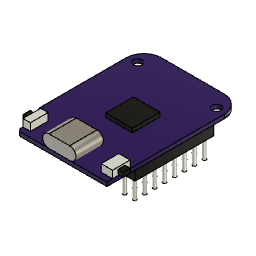
MLH1 v1.0 (Autodesk Fusion 360 archive; units mm, degrees)
design "ESP32-S2-mini"
Autodesk Fusion 360 part; units mm, degrees
sketch "Esquisse1" plane through (0, 0, 0) normal (0, 0, 1) x (1, 0, 0) in component "ESP32 S2-mini"
  line L0 (13.4, -16.1) -> (-11.6, -16.1)
  line L1 (-11.6, -16.1) -> (-11.6, 18.3)
  line L2 (-11.6, 18.3) -> (13.4, 18.3)
  line L3 (13.4, 18.3) -> (13.4, -16.1)
  line L4 (-11.6, -8.4281) -> (-9.4567, -9.7933)
  line L5 (-9.4567, -9.7933) -> (-9.4567, -15.5)
  line L6 (-9.4567, -15.5) -> (-8.8896, -16.1)
  circle A0 centre (-7.1, 13.8) radius 4.5
  circle A1 centre (8.9, 13.8) radius 4.5
  circle A2 centre (-9.1309, 14.2904) radius 1.122
  circle A3 centre (11.0247, 14.2904) radius 1.1083
  line L7 (-11.6, 11.162) -> (-6.6, 11.162)
  line L8 (-6.6, 11.162) -> (-6.6, -8.938)
  line L9 (-6.6, -8.938) -> (-11.6, -8.938)
  line L10 (-11.6, -8.938) -> (-11.6, 11.162)
  line L11 (13.4, 11.162) -> (8.4, 11.162)
  line L12 (8.4, 11.162) -> (8.4, -8.938)
  line L13 (8.4, -8.938) -> (13.4, -8.938)
  line L14 (13.4, -8.938) -> (13.4, 11.162)
  circle A4 centre (-10.5, 9.8) radius 0.4445
  circle A5 centre (-7.96, 9.8) radius 0.4445
  circle A6 centre (-10.5, 7.26) radius 0.4445
  circle A7 centre (-7.96, 7.26) radius 0.4445
  circle A8 centre (-10.5, 4.72) radius 0.4445
  circle A9 centre (-7.96, 4.72) radius 0.4445
  circle A10 centre (-10.5, 2.18) radius 0.4445
  circle A11 centre (-7.96, 2.18) radius 0.4445
  circle A12 centre (-10.5, -0.36) radius 0.4445
  circle A13 centre (-7.96, -0.36) radius 0.4445
  circle A14 centre (-10.5, -2.9) radius 0.4445
  circle A15 centre (-7.96, -2.9) radius 0.4445
  circle A16 centre (-10.5, -5.44) radius 0.4445
  circle A17 centre (-7.96, -5.44) radius 0.4445
  circle A18 centre (-10.5, -7.98) radius 0.4445
  circle A19 centre (-7.96, -7.98) radius 0.4445
  circle A20 centre (9.82, 9.8) radius 0.4445
  circle A21 centre (12.36, 9.8) radius 0.4445
  circle A22 centre (9.82, 7.26) radius 0.4445
  circle A23 centre (12.36, 7.26) radius 0.4445
  circle A24 centre (9.82, 4.72) radius 0.4445
  circle A25 centre (12.36, 4.72) radius 0.4445
  circle A26 centre (9.82, 2.18) radius 0.4445
  circle A27 centre (12.36, 2.18) radius 0.4445
  circle A28 centre (9.82, -0.36) radius 0.4445
  circle A29 centre (12.36, -0.36) radius 0.4445
  circle A30 centre (9.82, -2.9) radius 0.4445
  circle A31 centre (12.36, -2.9) radius 0.4445
  circle A32 centre (9.82, -5.44) radius 0.4445
  circle A33 centre (12.36, -5.44) radius 0.4445
  circle A34 centre (9.82, -7.98) radius 0.4445
  circle A35 centre (12.36, -7.98) radius 0.4445
  dimension "d1" = 25
  dimension "d2" = 34.4
  dimension "d3" = 4.5
  dimension "d4" = 4.5
  dimension "d7" = 5
  dimension "d8" = 20.1
  dimension "d9" = 5
  dimension "d10" = 20.1
  dimension "d36" = 0.889
  dimension "d39" = 2.54
  dimension "d40" = -17.78
  dimension "d41" = 8.5
  dimension "d42" = 1.1
  dimension "d43" = 0.889
  dimension "d44" = 8.5
  dimension "d45" = 20.32
  dimension "d48" = 2.54
  dimension "d49" = -17.78
  constraint horizontal L0
  constraint vertical L1
  constraint horizontal L2
  constraint vertical L3
  constraint coincident L1 L4.start
  constraint parallel L1 L5
  constraint coincident L0 L6.end
  constraint tangent L1 A0
  constraint tangent L2 A0
  constraint tangent L2 A1
  constraint tangent L3 A1
  constraint horizontal L7
  constraint vertical L8
  constraint horizontal L9
  constraint vertical L10
  constraint coincident L1 L7.start
  constraint horizontal L11
  constraint vertical L12
  constraint horizontal L13
  constraint vertical L14
  constraint coincident L3 L11.start
  measures "d1" distance of L0.start L0.end
  measures "d2" distance of L0.start L2.end
  measures "d3" radius of A0
  measures "d4" radius of A1
  measures "d7" distance of L7.start L7.end
  measures "d8" distance of L7.start L9.end
  measures "d9" distance of L11.start L11.end
  measures "d10" distance of L11.start L13.end
  measures "d36" diameter of A4
  measures "d41" distance of L2 A4.centre
  measures "d42" distance of L1 A4.centre
  measures "d43" diameter of A20
  measures "d44" distance of L2 A20.centre
  measures "d45" distance of A4.centre A20.centre
extrude "Extrusion1" add sketch "Esquisse1" along normal blind 1 contours L0 L2 L3 L4 L5 L6 A0 A1 L8 L9 L12 L13 | L3 A1 L11 L12 L13 L14 A20 | L3 A1 L11 | A1 L11 L12 | A1 L11 L12 A20 | L1 L4 A0 L7 L8 L9 L10 A5 | A1 A20 | A1 A20 | L1 A0 L7 | A0 L7 L8 | A0 L7 L8 A5 | A0 A5 | A0 A5 | A4 | A6 | A7 | A8 | A9 | A10 | A11 | A12 | A13 | A14 | A15 | A16 | A17 | A18 | A19 | A21 | A22 | A23 | A24 | A25 | A26 | A27 | A28 | A29 | A30 | A31 | A32 | A33 | A34 | A35 makes body 1 in component "ESP32 S2-mini"
extrude "Extrusion2" add sketch "Esquisse1" against normal blind 2.4 separate body contours L3 A1 L11 L12 L13 L14 A20 | A1 L11 L12 A20 | L1 L4 A0 L7 L8 L9 L10 A5 | A1 A20 | A1 A20 | A0 L7 L8 A5 | A0 A5 | A0 A5 | A4 | A6 | A7 | A8 | A9 | A10 | A11 | A12 | A13 | A14 | A15 | A16 | A17 | A18 | A19 | A21 | A22 | A23 | A24 | A25 | A26 | A27 | A28 | A29 | A30 | A31 | A32 | A33 | A34 | A35 makes body 2 at (-8.2667, -2.068, 0) makes body 3 at (10.0667, -2.238, 0) in component "ESP32 S2-mini"
sketch "Esquisse2" plane through (0, 0, 1) normal (0, 0, 1) x (-1, 0, 0) in component "ESP32 S2-mini"
  circle A0 centre (-11.0247, -14.2904) radius 1.1083
  circle A1 centre (9.1309, -14.2904) radius 1.122
  line L0 (-13.4, 16.1) -> (-13.4, -13.8)
  arc A2 (-13.4, -13.8) -> (-8.9, -18.3) centre (-8.9, -13.8) ccw
  line L1 (-8.9, -18.3) -> (7.1, -18.3)
  arc A3 (7.1, -18.3) -> (11.6, -13.8) centre (7.1, -13.8) ccw
  line L2 (11.6, -13.8) -> (11.6, 8.4281)
  line L3 (11.6, 8.4281) -> (9.4567, 9.7933)
  line L4 (9.4567, 9.7933) -> (9.4567, 15.5)
  line L5 (9.4567, 15.5) -> (8.8896, 16.1)
  line L6 (8.8896, 16.1) -> (-13.4, 16.1)
  line L7 (3.0077, 16.1) -> (-5.4923, 16.1)
  line L8 (-5.4923, 16.1) -> (-5.4923, 9.1)
  line L9 (-5.4923, 9.1) -> (3.0077, 9.1)
  line L10 (3.0077, 9.1) -> (3.0077, 16.1)
  line L11 (9.4567, 10.1759) -> (7.5567, 10.1759)
  line L12 (7.5567, 10.1759) -> (7.5567, 14.6759)
  line L13 (7.5567, 14.6759) -> (9.4567, 14.6759)
  line L14 (9.4567, 14.6759) -> (9.4567, 10.1759)
  line L15 (-13.4, 10.1759) -> (-10.5, 10.1759)
  line L16 (-10.5, 10.1759) -> (-10.5, 14.6759)
  line L17 (-10.5, 14.6759) -> (-13.4, 14.6759)
  line L18 (-13.4, 14.6759) -> (-13.4, 10.1759)
  line L19 (9.4567, 11.497) -> (10.8067, 11.497)
  line L20 (10.8067, 11.497) -> (10.8067, 13.297)
  line L21 (10.8067, 13.297) -> (9.4567, 13.297)
  line L22 (9.4567, 13.297) -> (9.4567, 11.497)
  line L23 (-13.4, 11.5) -> (-14.75, 11.5)
  line L24 (-14.75, 11.5) -> (-14.75, 13.3)
  line L25 (-14.75, 13.3) -> (-13.4, 13.3)
  line L26 (-13.4, 13.3) -> (-13.4, 11.5)
  line L27 (-5.7592, -5.0845) -> (1, -5.0845)
  line L28 (1, -5.0845) -> (1, 2)
  line L29 (1, 2) -> (-5.7592, 2)
  line L30 (-5.7592, 2) -> (-5.7592, -5.0845)
  dimension "d13" = 8.5
  dimension "d14" = 7
  dimension "d15" = 1.9
  dimension "d16" = 4.5
  dimension "d17" = 2.9
  dimension "d18" = 4.5
  dimension "d19" = 1.35
  dimension "d20" = 1.8
  dimension "d21" = 1.35
  dimension "d22" = 1.8
  constraint horizontal L7
  constraint vertical L8
  constraint horizontal L9
  constraint vertical L10
  constraint coincident L6 L7.start
  constraint horizontal L11
  constraint vertical L12
  constraint horizontal L13
  constraint vertical L14
  constraint coincident L4 L11.start
  constraint horizontal L15
  constraint vertical L16
  constraint horizontal L17
  constraint vertical L18
  constraint coincident L0 L15.start
  constraint horizontal L19
  constraint vertical L20
  constraint horizontal L21
  constraint vertical L22
  constraint coincident L14 L19.start
  constraint horizontal L23
  constraint vertical L24
  constraint horizontal L25
  constraint vertical L26
  constraint coincident L18 L23.start
  constraint horizontal L27
  constraint vertical L28
  constraint horizontal L29
  constraint vertical L30
  measures "d13" distance of L7.start L7.end
  measures "d14" distance of L7.start L9.end
  measures "d15" distance of L11.start L11.end
  measures "d16" distance of L11.start L13.end
  measures "d17" distance of L15.start L15.end
  measures "d18" distance of L15.start L17.end
  measures "d19" distance of L19.start L19.end
  measures "d20" distance of L19.start L21.end
  measures "d21" distance of L23.start L23.end
  measures "d22" distance of L23.start L25.end
extrude "Extrusion3" add sketch "Esquisse2" along normal blind 1.9 separate body contours L0 L15 L16 L17 L18 L26 | L4 L11 L12 L13 L14 L22 makes body 4 at (-9.4567, -13.1759, 2.2667) makes body 5 at (12.4333, -13.1759, 1) in component "ESP32 S2-mini"
extrude "Extrusion4" add sketch "Esquisse2" along normal blind 1.1 from surface at 0.3 separate body contours L0 L18 L23 L24 L25 L26 | L4 L14 L19 L20 L21 L22 makes body 6 at (14.3, -12.7, 1.3) makes body 7 at (-9.9067, -12.697, 1.3) in component "ESP32 S2-mini"
extrude "Extrusion5" add sketch "Esquisse2" along normal blind 1 separate body contours L27 L28 L29 L30 makes body 8 in component "ESP32 S2-mini"
extrude "Extrusion6" add sketch "Esquisse2" along normal blind 3.25 separate body contours L6 L7 L8 L9 L10 makes body 9 in component "ESP32 S2-mini"
sketch "Esquisse3" plane through (0, -16.1, 0) normal (0, -1, 0) x (1, 0, 0) in component "ESP32 S2-mini"
  line L0 (-3.0077, 1) -> (5.4923, 1)
  line L1 (5.4923, 1) -> (5.4923, 4.25)
  line L2 (5.4923, 4.25) -> (-3.0077, 4.25)
  line L3 (-3.0077, 4.25) -> (-3.0077, 1)
  circle A0 centre (-1.3777, 2.62) radius 1.63
  circle A1 centre (3.8623, 2.62) radius 1.63
  dimension "d32" = 1.63
  dimension "d33" = 1.63
  constraint tangent L3 A0
  constraint tangent L2 A0
  constraint tangent L1 A1
  constraint tangent L2 A1
  measures "d32" radius of A0
  measures "d33" radius of A1
extrude "Extrusion7" cut sketch "Esquisse3" against normal up to surface (7 mm away) contours L0 L3 A0 | L2 L3 A0 | L1 L2 A1 | L0 L1 A1 bodies 9 in component "ESP32 S2-mini"
extrude "Extrusion8" add sketch "Esquisse1" against normal blind 5 from surface at -2.4 separate body contours A1 A20 | A1 A20 | A0 A5 | A4 | A6 | A7 | A8 | A9 | A10 | A11 | A12 | A13 | A14 | A15 | A16 | A17 | A18 | A19 | A21 | A22 | A23 | A24 | A25 | A26 | A27 | A28 | A29 | A30 | A31 | A32 | A33 | A34 | A35 picked at (-7.979, 9.6771) makes body 10 at (12.8039, -5.4622, -5.7333) makes body 11 at (9.6996, 0.0679, -5.7333) makes body 12 at (12.8039, 4.6978, -5.7333) makes body 13 at (12.2396, 10.2279, -5.7333) makes body 14 at (-7.5161, 7.2378, -5.7333) makes body 15 at (-10.6204, 2.6079, -5.7333) makes body 16 at (-10.6204, -2.4721, -5.7333) makes body 17 at (-8.1016, -8.4014, -4.0667) makes body 18 at (-7.5161, -5.4622, -5.7333) makes body 19 at (-10.6204, 0.0679, -5.7333) makes body 20 at (-10.0561, 4.6978, -5.7333) makes body 21 at (-8.3291, 9.5524, -5.7333) makes body 22 at (10.2639, 7.2378, -5.7333) makes body 23 at (9.6996, 2.6079, -5.7333) makes body 24 at (9.6996, -2.4721, -5.7333) makes body 25 at (9.6784, -8.4014, -4.0667) makes body 26 at (10.2639, -5.4622, -5.7333) makes body 27 at (12.2396, 0.0679, -5.7333) makes body 28 at (10.2639, 4.6978, -5.7333) makes body 29 at (10.2623, 9.8443, -4.0667) makes body 30 at (-10.0561, 7.2378, -5.7333) makes body 31 at (-8.0804, 2.6079, -5.7333) makes body 32 at (-8.0804, -2.4721, -5.7333) makes body 33 at (-10.6416, -8.4014, -4.0667) makes body 34 at (-10.0561, -5.4622, -5.7333) makes body 35 at (-8.0804, 0.0679, -5.7333) makes body 36 at (-7.5161, 4.6978, -5.7333) makes body 37 at (-10.6204, 10.2279, -5.7333) makes body 38 at (12.8039, 7.2378, -5.7333) makes body 39 at (12.2396, 2.6079, -5.7333) makes body 40 at (12.2396, -2.4721, -5.7333) makes body 41 at (12.2184, -8.4014, -4.0667) in component "ESP32 S2-mini"
component "ESP32 S2-mini" placed x (1, 0, 0) y (0, 1, 0) z (0, 0, 1) at (0, 0, 0)
named bodies: "PCB", "J1", "J2", "RST", "B0", "RST bp", "B0 bp", "ESP32-S2", "ESB-C"

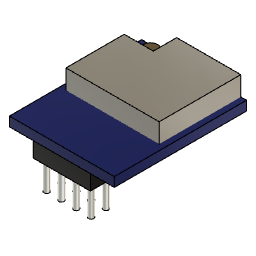
design "RA-02"
Autodesk Fusion 360 part; units mm, degrees
sketch "Esquisse1" plane through (0, 0, 0) normal (0, 0, 1) x (1, 0, 0) in component "LoRa RA-02"
  line L0 (0, 0) -> (18, 0)
  line L1 (18, 0) -> (18, -22.7)
  line L2 (18, -22.7) -> (0, -22.7)
  line L3 (0, -22.7) -> (0, 0)
  line L4 (1, 0) -> (17, 0)
  line L5 (17, 0) -> (17, -14)
  line L6 (17, -14) -> (1, -14)
  line L7 (1, -14) -> (1, 0)
  line L8 (13.9, -22.7) -> (4.1, -22.7)
  line L9 (4.1, -22.7) -> (4.1, -17.7)
  line L10 (4.1, -17.7) -> (13.9, -17.7)
  line L11 (13.9, -17.7) -> (13.9, -22.7)
  line L12 (1, 0) -> (6, 0)
  line L13 (6, 0) -> (6, -4)
  line L14 (6, -4) -> (1, -4)
  line L15 (1, -4) -> (1, 0)
  circle A0 centre (3.5142, -2) radius 1.25
  circle A1 centre (5.2, -21.5) radius 0.445
  circle A2 centre (7.74, -21.5) radius 0.445
  circle A3 centre (10.28, -21.5) radius 0.445
  circle A4 centre (12.82, -21.5) radius 0.445
  circle A5 centre (5.2, -18.96) radius 0.445
  circle A6 centre (7.74, -18.96) radius 0.445
  circle A7 centre (10.28, -18.96) radius 0.445
  circle A8 centre (12.82, -18.96) radius 0.445
  dimension "d1" = 18
  dimension "d2" = 22.7
  dimension "d3" = 16
  dimension "d4" = 14
  dimension "d5" = 9.8
  dimension "d6" = 5
  dimension "d7" = 5
  dimension "d8" = 4
  dimension "d9" = 2.5
  dimension "d18" = 0.89
  dimension "d21" = 7.62
  dimension "d22" = 2.54
  dimension "d23" = 1.2
  dimension "d24" = 1.1
  constraint horizontal L0
  constraint vertical L1
  constraint horizontal L2
  constraint vertical L3
  constraint coincident L0.start L3.end
  constraint horizontal L4
  constraint vertical L5
  constraint horizontal L6
  constraint vertical L7
  constraint coincident L0 L4.start
  constraint midpoint L0 L4
  constraint horizontal L8
  constraint vertical L9
  constraint horizontal L10
  constraint vertical L11
  constraint coincident L2 L8.start
  constraint midpoint L2 L8
  constraint horizontal L12
  constraint vertical L13
  constraint horizontal L14
  constraint vertical L15
  measures "d1" distance of L0.start L0.end
  measures "d2" distance of L0.start L2.end
  measures "d3" distance of L4.start L4.end
  measures "d4" distance of L4.start L6.end
  measures "d5" distance of L8.start L8.end
  measures "d6" distance of L8.start L10.end
  measures "d7" distance of L4.start L12.end
  measures "d8" distance of L4.start L14.end
  measures "d9" diameter of A0
  measures "d18" diameter of A1
  measures "d23" distance of L2 A1.centre
  measures "d24" distance of L9 A1.centre
extrude "Extrusion1" add sketch "Esquisse1" along normal blind 1.6 contours L0 L1 L2 L3 L5 L6 L7 L9 L10 L11 L15 | L0 L4 L7 L12 L13 L14 L15 | L0 L4 L5 L6 L7 L13 L14 | L2 L8 L9 L10 L11 | A0 | A1 | A2 | A3 | A4 | A5 | A6 | A7 | A8 makes body 1 in component "LoRa RA-02"
extrude "Extrusion2" add sketch "Esquisse1" against normal blind 2.6 separate body contours L2 L8 L9 L10 L11 | A1 | A2 | A3 | A4 | A5 | A6 | A7 | A8 makes body 2 in component "LoRa RA-02"
extrude "Extrusion3" add sketch "Esquisse1" along normal blind 4.9 separate body contours L0 L4 L5 L6 L7 L13 L14 makes body 3 in component "LoRa RA-02"
extrude "Extrusion4" add sketch "Esquisse1" along normal blind 3 separate body contours A0 makes body 4 in component "LoRa RA-02"
extrude "Extrusion5" add sketch "Esquisse1" against normal blind 5 from surface at -2.6 separate body contours A1 | A2 | A3 | A4 | A5 | A6 | A7 | A8 makes body 5 at (10.077, -19.356, -4.2667) makes body 6 at (8.1712, -21.6098, -5.9333) makes body 7 at (12.617, -21.896, -4.2667) makes body 8 at (8.1712, -19.0698, -5.9333) makes body 9 at (12.617, -19.356, -4.2667) makes body 10 at (5.6312, -21.6098, -5.9333) makes body 11 at (10.077, -21.896, -4.2667) makes body 12 at (5.6312, -19.0698, -5.9333) in component "LoRa RA-02"
component "LoRa RA-02" placed x (1, 0, 0) y (0, 1, 0) z (0, 0, 1) at (0, 0, 0)
named bodies: "PCB", "connecteur", "SX11278", "IPX"
